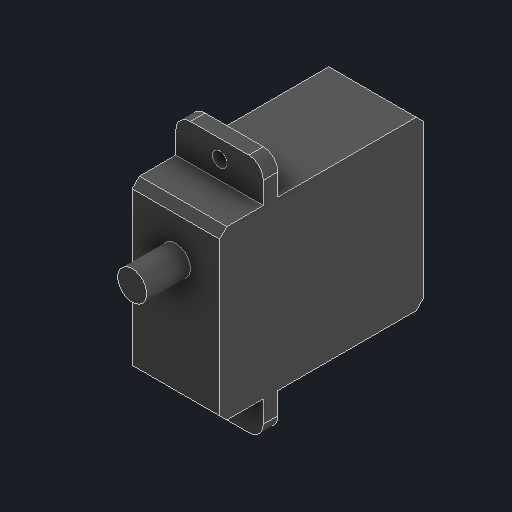
# Autodesk Inventor part: servo
Saved by Autodesk Inventor 2023 (Build 270158030, 158C)
## iProperties
Created: 2022-03-29
Part Number: servo
Material: Generic
Document SubType Name: Modeling
Designer: kardo
Density: 1 g/cm^3
Appearance: Dark Plastic
Author: kardo
Autodesk Inventor part; units mm, degrees
ref_plane "YZ Plane" through (0, 0, 0) normal (1, 0, 0) x (0, 1, 0)
ref_plane "XZ Plane" through (0, 0, 0) normal (0, 1, 0) x (-1, 0, 0)
ref_plane "XY Plane" through (0, 0, 0) normal (0, 0, 1) x (1, 0, 0)
derived "parameters_hardware.ipt"
sketch "sk_profile" plane through (0, 0, 0) normal (1, 0, 0) x (0, 1, 0)
  line L0 (0, 40.8) -> (0, -6.8) construction
  line L1 (-23.1, 0) -> (23.1, 0) construction
  line L2 (-11.5, 28) -> (11.5, 28)
  line L3 (11.5, 28) -> (11.5, 22)
  line L4 (11.5, 22) -> (16.5, 22)
  line L5 (-11.5, 28) -> (-11.5, 22)
  line L6 (-11.5, 22) -> (-16.5, 22)
  line L7 (-16.5, 22) -> (-16.5, 20)
  line L8 (-16.5, 20) -> (-11.5, 20)
  line L9 (-11.5, 20) -> (-11.5, 0)
  line L10 (16.5, 22) -> (16.5, 20)
  line L11 (16.5, 20) -> (11.5, 20)
  line L12 (11.5, 20) -> (11.5, 0)
  line L13 (-11.5, 0) -> (11.5, 0)
  line L14 (5, 28) -> (5, 34) construction
  point P0 (0, 0)
  dimension "d2" = 23
  dimension "d3" = 34
  dimension "d6" = 20
  dimension "d7" = 2
  dimension "d8" = 5
  dimension "d30" = 33
  constraints: 26 end point, 9 parallel, 4 collinear, 4 point on line, 2 equal length, 1 coincident, 1 other
  measures "d2" distance between parallel lines of L12 L9
  measures "d3" distance from line of L1 L14.end
  measures "d6" distance between parallel lines of L13 L8
  measures "d7" distance of L6.end L7.end
  measures "d8" distance between parallel lines of L14 L0
  measures "d30" distance between parallel lines of L10 L7
extrude "extrude_body" add sketch "sk_profile" along normal mid plane 12
sketch "sk_shaft" plane through (-6, -11.5, 28) normal (0, 0, 1) x (1, 0, 0)
  circle A0 centre (6, 16.5) radius 2
  point P0 (6, 11.5)
  dimension "d25" = 4
  constraints: 1 centre point, 1 coincident
  measures "d25" diameter of A0
extrude "extrude_shaft" add sketch "sk_shaft" along normal up to surface (6 mm away)
chamfer "chamfer_top" distance 1 angle 45 2 edges at (0, 11.5, 28) (0, -11.5, 28)
chamfer "chamfer_bottom" distance 1 angle 45 2 edges at (0, 11.5, 0) (0, -11.5, 0)
sketch "sk_drill" plane through (0, 0, 0) normal (0, 0, 1) x (1, 0, 0)
  line L0 (0, -19.6) -> (0, 19.6) construction
  line L1 (-19.6, 0) -> (19.6, 0) construction
  line L2 (0, -14) -> (0, 14) construction
  point P0 (0, 0)
  point P1 (0, 0)
  dimension "d17" = 28
  constraints: 2 coincident, 2 end point, 2 midpoint, 2 point on line
  measures "d17" distance of point (0, 14) point (0, -14)
hole "drill_pad" at (0, -14, 0) at (0, 14, 0) direction (0, 0, 1) diameter 2 end through all both
fillet "round_pads" radius 2 4 edges at (6, 16.5, 21) (-6, 16.5, 21) (6, -16.5, 21) (-6, -16.5, 21)
equation "\"d2\" = servo_length_body"
equation "\"d3\" = servo_height_joint"
equation "\"d6\" = servo_height_fastening"
equation "\"d8\" = servo_axis_location"
equation "\"d30\" = servo_length_fastening"
equation "\"d9\" = servo_width"
equation "\"d17\" = servo_fastening_distance"
equation "\"d18\" = servo_fastening_diam"
equation "\"servo_length_body\" = 23"
equation "\"servo_height_joint\" = 34"
equation "\"servo_height_fastening\" = 20"
equation "\"servo_axis_location\" = 5"
equation "\"servo_length_fastening\" = 33"
equation "\"servo_width\" = 12"
equation "\"servo_fastening_diam\" = 2"
equation "\"servo_fastening_distance\" = 28"
body "Solid1"
